Autodesk Inventor part; units mm, degrees
(part 2 of 2)
sketch "Sketch77" plane through (-48.732, -128.1414, 87.7359) normal (0, -0.819152, 0.5735764) x (1, 0, 0)
  line L0 (2.1727, -21.9196) -> (87.1828, -21.9196) construction
  line L1 (87.1828, -21.9196) -> (87.1828, -33.7509) construction
  line L2 (87.1828, -33.7509) -> (2.1727, -33.7509) construction
  line L3 (2.1727, -33.7509) -> (2.1727, -21.9196) construction
  spline S0 degree 2 poles (4.8848, -23.5103) (4.8848, -23.9277) (4.5464, -24.5996) (4.2624, -24.7873) knots 0 0 0 1 2 2 2
  spline S1 degree 2 poles (4.2624, -24.7873) (4.0302, -24.933) (3.5535, -25.0318) (3.183, -25.0318) knots 0 0 0 1 2 2 2
  line L4 (3.183, -25.0318) -> (2.4815, -25.0318)
  line L5 (2.4815, -25.0318) -> (2.4815, -21.9838)
  line L6 (2.4815, -21.9838) -> (3.1756, -21.9838)
  spline S2 degree 2 poles (3.1756, -21.9838) (3.6054, -21.9838) (4.0944, -22.1123) (4.2673, -22.2259) knots 0 0 0 1 2 2 2
  spline S3 degree 2 poles (4.2673, -22.2259) (4.5612, -22.421) (4.8848, -23.0657) (4.8848, -23.5103) knots 0 0 0 1 2 2 2
  spline S4 degree 2 poles (4.4624, -23.5053) (4.4624, -23.1546) (4.2303, -22.6581) (4.0006, -22.5173) knots 0 0 0 1 2 2 2
  spline S5 degree 2 poles (4.0006, -22.5173) (3.8375, -22.421) (3.4695, -22.3346) (3.1953, -22.3346) knots 0 0 0 1 2 2 2
  line L7 (3.1953, -22.3346) -> (2.8866, -22.3346)
  line L8 (2.8866, -22.3346) -> (2.8866, -24.6811)
  line L9 (2.8866, -24.6811) -> (3.1953, -24.6811)
  spline S6 degree 2 poles (3.1953, -24.6811) (3.4646, -24.6811) (3.8721, -24.5946) (4.0376, -24.4785) knots 0 0 0 1 2 2 2
  spline S7 degree 2 poles (4.0376, -24.4785) (4.25, -24.3353) (4.4624, -23.861) (4.4624, -23.5053) knots 0 0 0 1 2 2 2
  spline S8 degree 2 poles (6.3891, -25.096) (6.1198, -25.096) (5.7197, -24.9552) (5.5789, -24.8144) knots 0 0 0 1 2 2 2
  spline S9 degree 2 poles (5.5789, -24.8144) (5.4183, -24.6564) (5.2874, -24.2118) (5.2874, -23.8857) knots 0 0 0 1 2 2 2
  line L10 (5.2874, -23.8857) -> (5.2874, -21.9838)
  line L11 (5.2874, -21.9838) -> (5.6925, -21.9838)
  line L12 (5.6925, -21.9838) -> (5.6925, -23.8857)
  spline S10 degree 2 poles (5.6925, -23.8857) (5.6925, -24.0981) (5.7469, -24.3847) (5.8234, -24.5008) knots 0 0 0 1 2 2 2
  spline S11 degree 2 poles (5.8234, -24.5008) (5.9049, -24.6243) (6.1865, -24.7502) (6.3891, -24.7502) knots 0 0 0 1 2 2 2
  spline S12 degree 2 poles (6.3891, -24.7502) (6.5792, -24.7502) (6.8757, -24.6243) (6.9572, -24.5008) knots 0 0 0 1 2 2 2
  spline S13 degree 2 poles (6.9572, -24.5008) (7.0337, -24.3847) (7.0881, -24.1006) (7.0881, -23.8956) knots 0 0 0 1 2 2 2
  line L13 (7.0881, -23.8956) -> (7.0881, -21.9838)
  line L14 (7.0881, -21.9838) -> (7.4932, -21.9838)
  line L15 (7.4932, -21.9838) -> (7.4932, -23.8857)
  spline S14 degree 2 poles (7.4932, -23.8857) (7.4932, -24.2044) (7.3647, -24.6588) (7.2017, -24.8144) knots 0 0 0 1 2 2 2
  spline S15 degree 2 poles (7.2017, -24.8144) (7.056, -24.9577) (6.6706, -25.096) (6.3891, -25.096) knots 0 0 0 1 2 2 2
  line L16 (7.7451, -25.0318) -> (8.7726, -21.9838)
  line L17 (8.7726, -21.9838) -> (9.2716, -21.9838)
  line L18 (9.2716, -21.9838) -> (10.2991, -25.0318)
  line L19 (10.2991, -25.0318) -> (9.8718, -25.0318)
  line L20 (9.8718, -25.0318) -> (9.5951, -24.1797)
  line L21 (9.5951, -24.1797) -> (8.4318, -24.1797)
  line L22 (8.4318, -24.1797) -> (8.1551, -25.0318)
  line L23 (8.1551, -25.0318) -> (7.7451, -25.0318)
  line L24 (9.484, -23.8339) -> (9.0122, -22.3988)
  line L25 (9.0122, -22.3988) -> (8.5429, -23.8339)
  line L26 (8.5429, -23.8339) -> (9.484, -23.8339)
  line L27 (12.3541, -25.0318) -> (10.5881, -25.0318)
  line L28 (10.5881, -25.0318) -> (10.5881, -21.9838)
  line L29 (10.5881, -21.9838) -> (10.9932, -21.9838)
  line L30 (10.9932, -21.9838) -> (10.9932, -24.6712)
  line L31 (10.9932, -24.6712) -> (12.3541, -24.6712)
  line L32 (12.3541, -24.6712) -> (12.3541, -25.0318)
  line L33 (16.1926, -21.9838) -> (15.1428, -25.0318)
  line L34 (15.1428, -25.0318) -> (14.7056, -25.0318)
  line L35 (14.7056, -25.0318) -> (13.6558, -21.9838)
  line L36 (13.6558, -21.9838) -> (14.0906, -21.9838)
  line L37 (14.0906, -21.9838) -> (14.9353, -24.5156)
  line L38 (14.9353, -24.5156) -> (15.7801, -21.9838)
  line L39 (15.7801, -21.9838) -> (16.1926, -21.9838)
  line L40 (17.5461, -25.0318) -> (16.3655, -25.0318)
  line L41 (16.3655, -25.0318) -> (16.3655, -24.7206)
  line L42 (16.3655, -24.7206) -> (16.7532, -24.7206)
  line L43 (16.7532, -24.7206) -> (16.7532, -22.295)
  line L44 (16.7532, -22.295) -> (16.3655, -22.295)
  line L45 (16.3655, -22.295) -> (16.3655, -21.9838)
  line L46 (16.3655, -21.9838) -> (17.5461, -21.9838)
  line L47 (17.5461, -21.9838) -> (17.5461, -22.295)
  line L48 (17.5461, -22.295) -> (17.1583, -22.295)
  line L49 (17.1583, -22.295) -> (17.1583, -24.7206)
  line L50 (17.1583, -24.7206) -> (17.5461, -24.7206)
  line L51 (17.5461, -24.7206) -> (17.5461, -25.0318)
  spline S16 degree 2 poles (18.8972, -25.0862) (18.5662, -25.0862) (18.1019, -24.9478) (17.8969, -24.849) knots 0 0 0 1 2 2 2
  line L52 (17.8969, -24.849) -> (17.8969, -24.3402)
  line L53 (17.8969, -24.3402) -> (17.9265, -24.3402)
  spline S17 degree 2 poles (17.9265, -24.3402) (18.1266, -24.5279) (18.6329, -24.7354) (18.8676, -24.7354) knots 0 0 0 1 2 2 2
  spline S18 degree 2 poles (18.8676, -24.7354) (19.2035, -24.7354) (19.5468, -24.4563) (19.5468, -24.2266) knots 0 0 0 1 2 2 2
  spline S19 degree 2 poles (19.5468, -24.2266) (19.5468, -24.0438) (19.3665, -23.8166) (19.1714, -23.7598) knots 0 0 0 1 2 2 2
  spline S20 degree 2 poles (19.1714, -23.7598) (19.0306, -23.7202) (18.796, -23.6659) (18.6206, -23.6214) knots 0 0 0 1 2 2 2
  spline S21 degree 2 poles (18.6206, -23.6214) (18.4625, -23.5794) (18.213, -23.4535) (18.1167, -23.3522) knots 0 0 0 1 2 2 2
  spline S22 degree 2 poles (18.1167, -23.3522) (18.0228, -23.2509) (17.9191, -22.9792) (17.9191, -22.8014) knots 0 0 0 1 2 2 2
  spline S23 degree 2 poles (17.9191, -22.8014) (17.9191, -22.4309) (18.4971, -21.9295) (18.9442, -21.9295) knots 0 0 0 1 2 2 2
  spline S24 degree 2 poles (18.9442, -21.9295) (19.201, -21.9295) (19.6555, -22.0307) (19.8506, -22.1271) knots 0 0 0 1 2 2 2
  line L54 (19.8506, -22.1271) -> (19.8506, -22.6112)
  line L55 (19.8506, -22.6112) -> (19.821, -22.6112)
  spline S25 degree 2 poles (19.821, -22.6112) (19.6753, -22.4778) (19.2208, -22.2802) (18.9713, -22.2802) knots 0 0 0 1 2 2 2
  spline S26 degree 2 poles (18.9713, -22.2802) (18.6897, -22.2802) (18.3415, -22.5445) (18.3415, -22.7594) knots 0 0 0 1 2 2 2
  spline S27 degree 2 poles (18.3415, -22.7594) (18.3415, -22.9521) (18.5465, -23.1818) (18.7391, -23.2336) knots 0 0 0 1 2 2 2
  spline S28 degree 2 poles (18.7391, -23.2336) (18.8676, -23.2682) (19.2406, -23.3571) (19.3641, -23.3942) knots 0 0 0 1 2 2 2
  spline S29 degree 2 poles (19.3641, -23.3942) (19.6777, -23.4905) (19.9692, -23.8783) (19.9692, -24.1624) knots 0 0 0 1 2 2 2
  spline S30 degree 2 poles (19.9692, -24.1624) (19.9692, -24.3427) (19.8235, -24.6885) (19.6926, -24.8095) knots 0 0 0 1 2 2 2
  spline S31 degree 2 poles (19.6926, -24.8095) (19.5468, -24.9429) (19.1763, -25.0862) (18.8972, -25.0862) knots 0 0 0 1 2 2 2
  line L56 (21.4438, -25.0318) -> (20.2631, -25.0318)
  line L57 (20.2631, -25.0318) -> (20.2631, -24.7206)
  line L58 (20.2631, -24.7206) -> (20.6509, -24.7206)
  line L59 (20.6509, -24.7206) -> (20.6509, -22.295)
  line L60 (20.6509, -22.295) -> (20.2631, -22.295)
  line L61 (20.2631, -22.295) -> (20.2631, -21.9838)
  line L62 (20.2631, -21.9838) -> (21.4438, -21.9838)
  line L63 (21.4438, -21.9838) -> (21.4438, -22.295)
  line L64 (21.4438, -22.295) -> (21.056, -22.295)
  line L65 (21.056, -22.295) -> (21.056, -24.7206)
  line L66 (21.056, -24.7206) -> (21.4438, -24.7206)
  line L67 (21.4438, -24.7206) -> (21.4438, -25.0318)
  spline S32 degree 2 poles (24.1015, -22.3321) (24.2744, -22.5346) (24.4671, -23.1274) (24.4671, -23.5078) knots 0 0 0 1 2 2 2
  spline S33 degree 2 poles (24.4671, -23.5078) (24.4671, -23.8783) (24.2794, -24.4785) (24.1015, -24.6811) knots 0 0 0 1 2 2 2
  spline S34 degree 2 poles (24.1015, -24.6811) (23.9138, -24.8935) (23.4174, -25.096) (23.1185, -25.096) knots 0 0 0 1 2 2 2
  spline S35 degree 2 poles (23.1185, -25.096) (22.8097, -25.096) (22.3157, -24.8861) (22.1354, -24.6811) knots 0 0 0 1 2 2 2
  spline S36 degree 2 poles (22.1354, -24.6811) (21.96, -24.4785) (21.7723, -23.8833) (21.7723, -23.5078) knots 0 0 0 1 2 2 2
  spline S37 degree 2 poles (21.7723, -23.5078) (21.7723, -23.125) (21.9625, -22.542) (22.1379, -22.3321) knots 0 0 0 1 2 2 2
  spline S38 degree 2 poles (22.1379, -22.3321) (22.3157, -22.1295) (22.8122, -21.9196) (23.1185, -21.9196) knots 0 0 0 1 2 2 2
  spline S39 degree 2 poles (23.1185, -21.9196) (23.4297, -21.9196) (23.9286, -22.137) (24.1015, -22.3321) knots 0 0 0 1 2 2 2
  spline S40 degree 2 poles (24.0447, -23.5078) (24.0447, -23.2065) (23.9138, -22.7396) (23.7953, -22.5865) knots 0 0 0 1 2 2 2
  spline S41 degree 2 poles (23.7953, -22.5865) (23.6742, -22.4284) (23.3334, -22.2703) (23.1209, -22.2703) knots 0 0 0 1 2 2 2
  spline S42 degree 2 poles (23.1209, -22.2703) (22.9011, -22.2703) (22.5701, -22.4235) (22.4442, -22.5865) knots 0 0 0 1 2 2 2
  spline S43 degree 2 poles (22.4442, -22.5865) (22.3231, -22.7421) (22.1947, -23.2114) (22.1947, -23.5078) knots 0 0 0 1 2 2 2
  spline S44 degree 2 poles (22.1947, -23.5078) (22.1947, -24.108) (22.6986, -24.7453) (23.1209, -24.7453) knots 0 0 0 1 2 2 2
  spline S45 degree 2 poles (23.1209, -24.7453) (23.5433, -24.7453) (24.0447, -24.108) (24.0447, -23.5078) knots 0 0 0 1 2 2 2
  line L68 (27.0927, -25.0318) -> (26.6383, -25.0318)
  line L69 (26.6383, -25.0318) -> (25.2896, -22.4037)
  line L70 (25.2896, -22.4037) -> (25.2896, -25.0318)
  line L71 (25.2896, -25.0318) -> (24.9117, -25.0318)
  line L72 (24.9117, -25.0318) -> (24.9117, -21.9838)
  line L73 (24.9117, -21.9838) -> (25.4872, -21.9838)
  line L74 (25.4872, -21.9838) -> (26.7148, -24.397)
  line L75 (26.7148, -24.397) -> (26.7148, -21.9838)
  line L76 (26.7148, -21.9838) -> (27.0927, -21.9838)
  line L77 (27.0927, -21.9838) -> (27.0927, -25.0318)
  line L78 (30.7854, -25.0318) -> (29.0193, -25.0318)
  line L79 (29.0193, -25.0318) -> (29.0193, -21.9838)
  line L80 (29.0193, -21.9838) -> (29.4244, -21.9838)
  line L81 (29.4244, -21.9838) -> (29.4244, -24.6712)
  line L82 (29.4244, -24.6712) -> (30.7854, -24.6712)
  line L83 (30.7854, -24.6712) -> (30.7854, -25.0318)
  line L84 (32.1661, -25.0318) -> (30.9855, -25.0318)
  line L85 (30.9855, -25.0318) -> (30.9855, -24.7206)
  line L86 (30.9855, -24.7206) -> (31.3733, -24.7206)
  line L87 (31.3733, -24.7206) -> (31.3733, -22.295)
  line L88 (31.3733, -22.295) -> (30.9855, -22.295)
  line L89 (30.9855, -22.295) -> (30.9855, -21.9838)
  line L90 (30.9855, -21.9838) -> (32.1661, -21.9838)
  line L91 (32.1661, -21.9838) -> (32.1661, -22.295)
  line L92 (32.1661, -22.295) -> (31.7784, -22.295)
  line L93 (31.7784, -22.295) -> (31.7784, -24.7206)
  line L94 (31.7784, -24.7206) -> (32.1661, -24.7206)
  line L95 (32.1661, -24.7206) -> (32.1661, -25.0318)
  spline S46 degree 2 poles (35.0709, -23.5103) (35.0709, -23.9277) (34.7325, -24.5996) (34.4484, -24.7873) knots 0 0 0 1 2 2 2
  spline S47 degree 2 poles (34.4484, -24.7873) (34.2163, -24.933) (33.7395, -25.0318) (33.369, -25.0318) knots 0 0 0 1 2 2 2
  line L96 (33.369, -25.0318) -> (32.6676, -25.0318)
  line L97 (32.6676, -25.0318) -> (32.6676, -21.9838)
  line L98 (32.6676, -21.9838) -> (33.3616, -21.9838)
  spline S48 degree 2 poles (33.3616, -21.9838) (33.7914, -21.9838) (34.2805, -22.1123) (34.4534, -22.2259) knots 0 0 0 1 2 2 2
  spline S49 degree 2 poles (34.4534, -22.2259) (34.7473, -22.421) (35.0709, -23.0657) (35.0709, -23.5103) knots 0 0 0 1 2 2 2
  spline S50 degree 2 poles (34.6485, -23.5053) (34.6485, -23.1546) (34.4163, -22.6581) (34.1866, -22.5173) knots 0 0 0 1 2 2 2
  spline S51 degree 2 poles (34.1866, -22.5173) (34.0236, -22.421) (33.6556, -22.3346) (33.3814, -22.3346) knots 0 0 0 1 2 2 2
  line L99 (33.3814, -22.3346) -> (33.0726, -22.3346)
  line L100 (33.0726, -22.3346) -> (33.0726, -24.6811)
  line L101 (33.0726, -24.6811) -> (33.3814, -24.6811)
  spline S52 degree 2 poles (33.3814, -24.6811) (33.6506, -24.6811) (34.0582, -24.5946) (34.2237, -24.4785) knots 0 0 0 1 2 2 2
  spline S53 degree 2 poles (34.2237, -24.4785) (34.4361, -24.3353) (34.6485, -23.861) (34.6485, -23.5053) knots 0 0 0 1 2 2 2
  line L102 (4.3093, -27.4592) -> (2.9903, -30.0503)
  line L103 (2.9903, -30.0503) -> (2.5556, -30.0503)
  line L104 (2.5556, -30.0503) -> (3.9487, -27.3604)
  line L105 (3.9487, -27.3604) -> (2.3753, -27.3604)
  line L106 (2.3753, -27.3604) -> (2.3753, -27.0023)
  line L107 (2.3753, -27.0023) -> (4.3093, -27.0023)
  line L108 (4.3093, -27.0023) -> (4.3093, -27.4592)
  line L109 (5.3368, -30.0503) -> (4.8478, -30.0503)
  line L110 (4.8478, -30.0503) -> (4.8478, -29.4673)
  line L111 (4.8478, -29.4673) -> (5.3368, -29.4673)
  line L112 (5.3368, -29.4673) -> (5.3368, -30.0503)
  line L113 (7.8315, -30.0503) -> (5.9519, -30.0503)
  line L114 (5.9519, -30.0503) -> (5.9519, -29.618)
  spline S54 degree 2 poles (5.9519, -29.618) (6.1544, -29.4278) (6.515, -29.0746) (6.6879, -28.8844) knots 0 0 0 1 2 2 2
  spline S55 degree 2 poles (6.6879, -28.8844) (7.0362, -28.5016) (7.2906, -28.0421) (7.2906, -27.7976) knots 0 0 0 1 2 2 2
  spline S56 degree 2 poles (7.2906, -27.7976) (7.2906, -27.6692) (7.2116, -27.4765) (7.1399, -27.4148) knots 0 0 0 1 2 2 2
  spline S57 degree 2 poles (7.1399, -27.4148) (7.0683, -27.353) (6.8806, -27.2913) (6.767, -27.2913) knots 0 0 0 1 2 2 2
  spline S58 degree 2 poles (6.767, -27.2913) (6.6583, -27.2913) (6.436, -27.3456) (6.3347, -27.3876) knots 0 0 0 1 2 2 2
  spline S59 degree 2 poles (6.3347, -27.3876) (6.2483, -27.4222) (6.0877, -27.521) (6.0383, -27.5555) knots 0 0 0 1 2 2 2
  line L115 (6.0383, -27.5555) -> (6.0161, -27.5555)
  line L116 (6.0161, -27.5555) -> (6.0161, -27.1208)
  spline S60 degree 2 poles (6.0161, -27.1208) (6.1421, -27.0591) (6.5941, -26.938) (6.7966, -26.938) knots 0 0 0 1 2 2 2
  spline S61 degree 2 poles (6.7966, -26.938) (7.2239, -26.938) (7.7056, -27.3901) (7.7056, -27.7754) knots 0 0 0 1 2 2 2
  spline S62 degree 2 poles (7.7056, -27.7754) (7.7056, -27.9557) (7.6216, -28.257) (7.5475, -28.3855) knots 0 0 0 1 2 2 2
  spline S63 degree 2 poles (7.5475, -28.3855) (7.4734, -28.5189) (7.2585, -28.7807) (7.1399, -28.9066) knots 0 0 0 1 2 2 2
  spline S64 degree 2 poles (7.1399, -28.9066) (6.9473, -29.1166) (6.4755, -29.5661) (6.3347, -29.697) knots 0 0 0 1 2 2 2
  line L117 (6.3347, -29.697) -> (7.8315, -29.697)
  line L118 (7.8315, -29.697) -> (7.8315, -30.0503)
  spline S65 degree 2 poles (10.0867, -29.082) (10.0867, -29.3018) (9.9459, -29.6773) (9.8174, -29.8156) knots 0 0 0 1 2 2 2
  spline S66 degree 2 poles (9.8174, -29.8156) (9.689, -29.9539) (9.3061, -30.1145) (9.069, -30.1145) knots 0 0 0 1 2 2 2
  spline S67 degree 2 poles (9.069, -30.1145) (8.8517, -30.1145) (8.4268, -30.0182) (8.2712, -29.9416) knots 0 0 0 1 2 2 2
  line L119 (8.2712, -29.9416) -> (8.2712, -29.5093)
  line L120 (8.2712, -29.5093) -> (8.3009, -29.5093)
  spline S68 degree 2 poles (8.3009, -29.5093) (8.3478, -29.5439) (8.5232, -29.6328) (8.6294, -29.6723) knots 0 0 0 1 2 2 2
  spline S69 degree 2 poles (8.6294, -29.6723) (8.7504, -29.7143) (8.9505, -29.7613) (9.0764, -29.7613) knots 0 0 0 1 2 2 2
  spline S70 degree 2 poles (9.0764, -29.7613) (9.1999, -29.7613) (9.4321, -29.6723) (9.5161, -29.576) knots 0 0 0 1 2 2 2
  spline S71 degree 2 poles (9.5161, -29.576) (9.5927, -29.4846) (9.6717, -29.2426) (9.6717, -29.0795) knots 0 0 0 1 2 2 2
  spline S72 degree 2 poles (9.6717, -29.0795) (9.6717, -28.9165) (9.5828, -28.709) (9.4988, -28.6399) knots 0 0 0 1 2 2 2
  spline S73 degree 2 poles (9.4988, -28.6399) (9.4124, -28.5633) (9.1555, -28.4991) (8.9999, -28.4991) knots 0 0 0 1 2 2 2
  spline S74 degree 2 poles (8.9999, -28.4991) (8.8319, -28.4991) (8.4985, -28.551) (8.3972, -28.5732) knots 0 0 0 1 2 2 2
  line L121 (8.3972, -28.5732) -> (8.3972, -27.0023)
  line L122 (8.3972, -27.0023) -> (10.0694, -27.0023)
  line L123 (10.0694, -27.0023) -> (10.0694, -27.3604)
  line L124 (10.0694, -27.3604) -> (8.7899, -27.3604)
  line L125 (8.7899, -27.3604) -> (8.7899, -28.173)
  spline S75 degree 2 poles (8.7899, -28.173) (8.864, -28.1632) (9.0073, -28.1558) (9.0666, -28.1558) knots 0 0 0 1 2 2 2
  spline S76 degree 2 poles (9.0666, -28.1558) (9.3012, -28.1558) (9.6248, -28.2323) (9.773, -28.346) knots 0 0 0 1 2 2 2
  spline S77 degree 2 poles (9.773, -28.346) (9.9237, -28.4596) (10.0867, -28.8054) (10.0867, -29.082) knots 0 0 0 1 2 2 2
  line L126 (11.1809, -30.0503) -> (10.6918, -30.0503)
  line L127 (10.6918, -30.0503) -> (10.6918, -29.4673)
  line L128 (10.6918, -29.4673) -> (11.1809, -29.4673)
  line L129 (11.1809, -29.4673) -> (11.1809, -30.0503)
  line L130 (13.6756, -30.0503) -> (11.7959, -30.0503)
  line L131 (11.7959, -30.0503) -> (11.7959, -29.618)
  spline S78 degree 2 poles (11.7959, -29.618) (11.9985, -29.4278) (12.3591, -29.0746) (12.532, -28.8844) knots 0 0 0 1 2 2 2
  spline S79 degree 2 poles (12.532, -28.8844) (12.8803, -28.5016) (13.1347, -28.0421) (13.1347, -27.7976) knots 0 0 0 1 2 2 2
  spline S80 degree 2 poles (13.1347, -27.7976) (13.1347, -27.6692) (13.0556, -27.4765) (12.984, -27.4148) knots 0 0 0 1 2 2 2
  spline S81 degree 2 poles (12.984, -27.4148) (12.9124, -27.353) (12.7247, -27.2913) (12.611, -27.2913) knots 0 0 0 1 2 2 2
  spline S82 degree 2 poles (12.611, -27.2913) (12.5023, -27.2913) (12.28, -27.3456) (12.1788, -27.3876) knots 0 0 0 1 2 2 2
  spline S83 degree 2 poles (12.1788, -27.3876) (12.0923, -27.4222) (11.9318, -27.521) (11.8824, -27.5555) knots 0 0 0 1 2 2 2
  line L132 (11.8824, -27.5555) -> (11.8601, -27.5555)
  line L133 (11.8601, -27.5555) -> (11.8601, -27.1208)
  spline S84 degree 2 poles (11.8601, -27.1208) (11.9861, -27.0591) (12.4381, -26.938) (12.6407, -26.938) knots 0 0 0 1 2 2 2
  spline S85 degree 2 poles (12.6407, -26.938) (13.068, -26.938) (13.5496, -27.3901) (13.5496, -27.7754) knots 0 0 0 1 2 2 2
  spline S86 degree 2 poles (13.5496, -27.7754) (13.5496, -27.9557) (13.4657, -28.257) (13.3916, -28.3855) knots 0 0 0 1 2 2 2
  spline S87 degree 2 poles (13.3916, -28.3855) (13.3175, -28.5189) (13.1026, -28.7807) (12.984, -28.9066) knots 0 0 0 1 2 2 2
  spline S88 degree 2 poles (12.984, -28.9066) (12.7913, -29.1166) (12.3196, -29.5661) (12.1788, -29.697) knots 0 0 0 1 2 2 2
  line L134 (12.1788, -29.697) -> (13.6756, -29.697)
  line L135 (13.6756, -29.697) -> (13.6756, -30.0503)
  spline S89 degree 2 poles (15.9307, -29.082) (15.9307, -29.3018) (15.7899, -29.6773) (15.6615, -29.8156) knots 0 0 0 1 2 2 2
  spline S90 degree 2 poles (15.6615, -29.8156) (15.5331, -29.9539) (15.1502, -30.1145) (14.9131, -30.1145) knots 0 0 0 1 2 2 2
  spline S91 degree 2 poles (14.9131, -30.1145) (14.6957, -30.1145) (14.2709, -30.0182) (14.1153, -29.9416) knots 0 0 0 1 2 2 2
  line L136 (14.1153, -29.9416) -> (14.1153, -29.5093)
  line L137 (14.1153, -29.5093) -> (14.1449, -29.5093)
  spline S92 degree 2 poles (14.1449, -29.5093) (14.1918, -29.5439) (14.3672, -29.6328) (14.4734, -29.6723) knots 0 0 0 1 2 2 2
  spline S93 degree 2 poles (14.4734, -29.6723) (14.5945, -29.7143) (14.7945, -29.7613) (14.9205, -29.7613) knots 0 0 0 1 2 2 2
  spline S94 degree 2 poles (14.9205, -29.7613) (15.044, -29.7613) (15.2762, -29.6723) (15.3602, -29.576) knots 0 0 0 1 2 2 2
  spline S95 degree 2 poles (15.3602, -29.576) (15.4367, -29.4846) (15.5158, -29.2426) (15.5158, -29.0795) knots 0 0 0 1 2 2 2
  spline S96 degree 2 poles (15.5158, -29.0795) (15.5158, -28.9165) (15.4268, -28.709) (15.3429, -28.6399) knots 0 0 0 1 2 2 2
  spline S97 degree 2 poles (15.3429, -28.6399) (15.2564, -28.5633) (14.9995, -28.4991) (14.8439, -28.4991) knots 0 0 0 1 2 2 2
  spline S98 degree 2 poles (14.8439, -28.4991) (14.676, -28.4991) (14.3425, -28.551) (14.2412, -28.5732) knots 0 0 0 1 2 2 2
  line L138 (14.2412, -28.5732) -> (14.2412, -27.0023)
  line L139 (14.2412, -27.0023) -> (15.9134, -27.0023)
  line L140 (15.9134, -27.0023) -> (15.9134, -27.3604)
  line L141 (15.9134, -27.3604) -> (14.634, -27.3604)
  line L142 (14.634, -27.3604) -> (14.634, -28.173)
  spline S99 degree 2 poles (14.634, -28.173) (14.7081, -28.1632) (14.8513, -28.1558) (14.9106, -28.1558) knots 0 0 0 1 2 2 2
  spline S100 degree 2 poles (14.9106, -28.1558) (15.1453, -28.1558) (15.4688, -28.2323) (15.617, -28.346) knots 0 0 0 1 2 2 2
  spline S101 degree 2 poles (15.617, -28.346) (15.7677, -28.4596) (15.9307, -28.8054) (15.9307, -29.082) knots 0 0 0 1 2 2 2
  point P0 (48.732, 1.6298)
  constraints: 2 other
extrude "Extrusion66" add sketch "Sketch77" along normal blind 1
body "Solid1"
